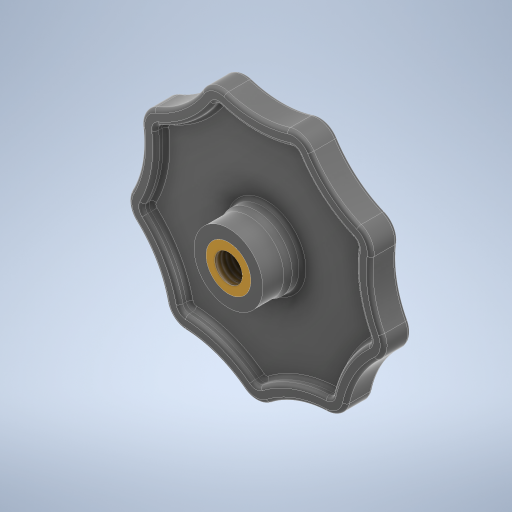
# Autodesk Inventor part: Bed Knob
Saved by Autodesk Inventor 2024 (Build 280153000, 153)
## iProperties
Created: 2024-12-30
Part Number: Bed Knob
Material: ABS Plastic
Document SubType Name: Modeling
Designer: Ishaan
Density: 1.06 g/cm^3
Appearance: Smooth - Black
Author: Ishaan
Autodesk Inventor part; units mm, degrees
ref_plane "YZ Plane" through (0, 0, 0) normal (1, 0, 0) x (0, 1, 0)
ref_plane "XZ Plane" through (0, 0, 0) normal (0, 1, 0) x (-1, 0, 0)
ref_plane "XY Plane" through (0, 0, 0) normal (0, 0, 1) x (1, 0, 0)
sketch "Sketch1" plane through (0, 0, 0) normal (0, 0, 1) x (1, 0, 0)
  circle A0 centre (0, 0) radius 20
  dimension "d0" = 40
  constraints: 1 centre point, 1 coincident
  measures "d0" diameter of A0
extrude "Extrusion1" add sketch "Sketch1" along normal mid plane 4
sketch "Sketch2" plane through (0, 0, 2) normal (0, 0, 1) x (1, 0, 0)
  circle A0 centre (0, 0) radius 5
  dimension "d3" = 10
  constraints: 1 centre point, 1 coincident
  measures "d3" diameter of A0
extrude "Extrusion2" add sketch "Sketch2" along normal blind 4
sketch "Sketch3" plane through (0, 0, 2) normal (0, 0, 1) x (1, 0, 0)
  circle A0 centre (0, 32) radius 15
  point P0 (0, 0)
  dimension "d6" = 30
  dimension "d7" = 32
  constraints: 1 centre point, 1 vertical alignment
  measures "d6" diameter of A0
  measures "d7" distance of A0.centre point (0, 0)
extrude "Extrusion3" cut sketch "Sketch3" against normal through all
pattern_circular "Circular Pattern1" count 9 over 360 about axis through (0, 0, 2) along (0, 0, 1) of "Extrusion3"
fillet "Fillet1" radius 3 9 edges at (17.1583, 9.9064, 0) (6.7764, 18.6179, 0) (-6.7764, 18.6179, 0) (-17.1583, 9.9064, 0) (-19.5117, -3.4404, 0) (-12.7354, -15.1774, 0) (0, -19.8127, 0) (12.7354, -15.1774, 0) (19.5117, -3.4404, 0)
sketch "Sketch4" plane through (0, 0, 6) normal (0, 0, 1) x (1, 0, 0)
  circle A0 centre (0, 0) radius 3.25
  dimension "d15" = 6.5
  constraints: 1 centre point, 1 coincident
  measures "d15" diameter of A0
extrude "Extrusion4" cut sketch "Sketch4" against normal through all
sketch "Sketch5" plane through (0, 0, 6) normal (0, 0, 1) x (1, 0, 0)
  circle A0 centre (0, 0) radius 3.25 projected
  circle A1 centre (0, 0) radius 2
  dimension "d18" = 4
  constraints: 1 centre point, 1 coincident
  measures "d18" diameter of A1
extrude "Extrusion5" add sketch "Sketch5" against normal up to surface (8 mm away) separate body
thread "Thread1" size "M4x0.7" class "6H" standard "ANSI Metric M Profile" length 10
sketch "Sketch6" plane through (0, 0, -2) normal (0, 0, -1) x (-1, 0, 0)
  circle A0 centre (0, 0) radius 3.25 projected
  arc A1 (-18.2024, -1.3573) -> (-17.5689, -4.9501) centre (-15.5401, -2.7401) ccw projected
  arc A2 (-13.0713, -12.74) -> (-17.5689, -4.9501) centre (-27.7128, -16) ccw projected
  arc A3 (-13.0713, -12.74) -> (-10.2767, -15.085) centre (-10.1431, -12.088) ccw projected
  arc A4 (-1.8241, -18.1615) -> (-10.2767, -15.085) centre (-10.9446, -30.0702) ccw projected
  arc A5 (-1.8241, -18.1615) -> (1.8241, -18.1615) centre (0, -15.7798) ccw projected
  arc A6 (10.2767, -15.085) -> (1.8241, -18.1615) centre (10.9446, -30.0702) ccw projected
  arc A7 (10.2767, -15.085) -> (13.0713, -12.74) centre (10.1431, -12.088) ccw projected
  arc A8 (17.5689, -4.9501) -> (13.0713, -12.74) centre (27.7128, -16) ccw projected
  arc A9 (17.5689, -4.9501) -> (18.2024, -1.3573) centre (15.5401, -2.7401) ccw projected
  arc A10 (16.6404, 7.501) -> (18.2024, -1.3573) centre (31.5138, 5.5567) ccw projected
  arc A11 (16.6404, 7.501) -> (14.8163, 10.6605) centre (13.6657, 7.8899) ccw projected
  arc A12 (7.9257, 16.4424) -> (14.8163, 10.6605) centre (20.5692, 24.5134) ccw projected
  arc A13 (7.9257, 16.4424) -> (4.4975, 17.6901) centre (5.397, 14.8282) ccw projected
  arc A14 (-4.4975, 17.6901) -> (4.4975, 17.6901) centre (0, 32) ccw projected
  arc A15 (-4.4975, 17.6901) -> (-7.9257, 16.4424) centre (-5.397, 14.8282) ccw projected
  arc A16 (-14.8163, 10.6605) -> (-7.9257, 16.4424) centre (-20.5692, 24.5134) ccw projected
  arc A17 (-14.8163, 10.6605) -> (-16.6404, 7.501) centre (-13.6657, 7.8899) ccw projected
  arc A18 (-18.2024, -1.3573) -> (-16.6404, 7.501) centre (-31.5138, 5.5567) ccw projected
  arc A19 (-11.1192, -12.3054) -> (-10.1876, -13.087) centre (-10.1431, -12.088) ccw
  arc A20 (-11.1192, -12.3054) -> (-16.2163, -3.4768) centre (-27.7128, -16) ccw
  arc A21 (-16.4275, -2.2792) -> (-16.2163, -3.4768) centre (-15.5401, -2.7401) ccw
  arc A22 (-16.4275, -2.2792) -> (-14.6573, 7.7603) centre (-31.5138, 5.5567) ccw
  arc A23 (-14.0492, 8.8134) -> (-14.6573, 7.7603) centre (-13.6657, 7.8899) ccw
  arc A24 (-14.0492, 8.8134) -> (-6.2399, 15.3662) centre (-20.5692, 24.5134) ccw
  arc A25 (-5.0972, 15.7821) -> (-6.2399, 15.3662) centre (-5.397, 14.8282) ccw
  arc A26 (-5.0972, 15.7821) -> (5.0972, 15.7821) centre (0, 32) ccw
  arc A27 (6.2399, 15.3662) -> (5.0972, 15.7821) centre (5.397, 14.8282) ccw
  arc A28 (6.2399, 15.3662) -> (14.0492, 8.8134) centre (20.5692, 24.5134) ccw
  arc A29 (14.6573, 7.7603) -> (14.0492, 8.8134) centre (13.6657, 7.8899) ccw
  arc A30 (14.6573, 7.7603) -> (16.4275, -2.2792) centre (31.5138, 5.5567) ccw
  arc A31 (16.2163, -3.4768) -> (16.4275, -2.2792) centre (15.5401, -2.7401) ccw
  arc A32 (16.2163, -3.4768) -> (11.1192, -12.3054) centre (27.7128, -16) ccw
  arc A33 (10.1876, -13.087) -> (11.1192, -12.3054) centre (10.1431, -12.088) ccw
  arc A34 (10.1876, -13.087) -> (0.608, -16.5737) centre (10.9446, -30.0702) ccw
  arc A35 (-0.608, -16.5737) -> (0.608, -16.5737) centre (0, -15.7798) ccw
  arc A36 (-0.608, -16.5737) -> (-10.1876, -13.087) centre (-10.9446, -30.0702) ccw
  circle A37 centre (0, 0) radius 5.25
  dimension "d23" = 2
  dimension "d24" = 2
  constraints: 36 point on circle, 19 centre point, 17 other
  measures "d23" radial gap between concentric circles of A4 A36
  measures "d24" radial gap between concentric circles of A0 A37
extrude "Extrusion6" cut sketch "Sketch6" against normal blind 1.5 contours A20 A21 A22 A23 A24 A25 A26 A27 A28 A29 A30 A31 A32 A33 A34 A35 A36 A19 bodies 1
mirror "Mirror1" about plane through (0, 0, 0) normal (0, 0, 1) of "Extrusion6" bodies 1
fillet "Fillet3" radius 2 1 edges at (-5, 0, 2)
fillet "Fillet4" radius 0.5 111 edges at (16.5249, -2.9138, 2) (12.9904, -7.5, 2) (10.7858, -12.8541, 2) (5.1303, -14.0954, 2) (0, -16.7798, 2) (-5.1303, -14.0954, 2) (-10.7858, -12.8541, 2) (-12.9904, -7.5, 2) (-16.5249, -2.9138, 2) (-14.7721, 2.6047, 2) (-14.5317, 8.3899, 2) (-9.6418, 11.4907, 2) (-5.739, 15.7678, 2) (0, 15, 2) (5.739, 15.7678, 2) (9.6418, 11.4907, 2) (14.5317, 8.3899, 2) (14.7721, 2.6047, 2) (14.5317, 8.3899, 0.5) (9.6418, 11.4907, 0.5) (5.739, 15.7678, 0.5) (0, 15, 0.5) (-5.739, 15.7678, 0.5) (-9.6418, 11.4907, 0.5) (-14.5317, 8.3899, 0.5) (-14.7721, 2.6047, 0.5) (-16.5249, -2.9138, 0.5) (-12.9904, -7.5, 0.5) (-10.7858, -12.8541, 0.5) (-5.1303, -14.0954, 0.5) (0, -16.7798, 0.5) (5.1303, -14.0954, 0.5) (10.7858, -12.8541, 0.5) (12.9904, -7.5, 0.5) (16.5249, -2.9138, 0.5) (14.7721, 2.6047, 0.5) (5.25, 0, -0.5) (5.25, 0, 0.5) (-6.423, 17.6472, 2) (-10.9274, 13.0228, 2) (-16.2638, 9.3899, 2) (-16.7417, 2.952, 2) (-18.4945, -3.2611, 2) (-14.7224, -8.5, 2) (-12.0714, -14.3861, 2) (-5.8143, -15.9748, 2) (0, -18.7798, 2) (5.8143, -15.9748, 2) (12.0714, -14.3862, 2) (14.7224, -8.5, 2) (18.4945, -3.2611, 2) (16.7417, 2.952, 2) (16.2638, 9.3899, 2) (10.9274, 13.0228, 2) (6.423, 17.6472, 2) (0, 17, 2) (6.423, 17.6472, -2) (10.9274, 13.0228, -2) (16.2638, 9.3899, -2) (16.7417, 2.952, -2) (18.4945, -3.2611, -2) (14.7224, -8.5, -2) (12.0714, -14.3862, -2) (5.8143, -15.9748, -2) (0, -18.7798, -2) (-5.8143, -15.9748, -2) (-12.0714, -14.3861, -2) (-14.7224, -8.5, -2) (-18.4945, -3.2611, -2) (-16.7417, 2.952, -2) (-16.2638, 9.3899, -2) (-10.9274, 13.0228, -2) (-6.423, 17.6472, -2) (0, 17, -2) (5.739, 15.7678, -0.5) (0, 15, -0.5) (-5.739, 15.7678, -0.5) (-9.6418, 11.4907, -0.5) (-14.5317, 8.3899, -0.5) (-14.7721, 2.6047, -0.5) (-16.5249, -2.9138, -0.5) (-12.9904, -7.5, -0.5) (-10.7858, -12.8541, -0.5) (-5.1303, -14.0954, -0.5) (0, -16.7798, -0.5) (5.1303, -14.0954, -0.5) (10.7858, -12.8541, -0.5) (12.9904, -7.5, -0.5) (16.5249, -2.9138, -0.5) (14.7721, 2.6047, -0.5) (14.5317, 8.3899, -0.5) (9.6418, 11.4907, -0.5) (5.25, 0, -2) (5.739, 15.7678, -2) (0, 15, -2) (-5.739, 15.7678, -2) (-9.6418, 11.4907, -2) (-14.5317, 8.3899, -2) (-14.7721, 2.6047, -2) (-16.5249, -2.9138, -2) (-12.9904, -7.5, -2) (-10.7858, -12.8541, -2) (-5.1303, -14.0954, -2) (0, -16.7798, -2) (5.1303, -14.0954, -2) (10.7858, -12.8541, -2) (12.9904, -7.5, -2) (16.5249, -2.9138, -2) (14.7721, 2.6047, -2) (14.5317, 8.3899, -2) (9.6418, 11.4907, -2)
body "Solid1"
body "Solid2"
